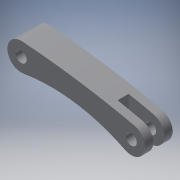
# Autodesk Inventor part: legA_mini
Saved by Autodesk Inventor 2017 (Build 210142000, 142)
## iProperties
Created: 2016-08-26
Part Number: legA_mini
Material: Generic
Document SubType Name: Modeling
Designer: Nic
Density: 1 g/cm^3
Appearance: Default
Author: Nic
Autodesk Inventor part; units mm, degrees
ref_plane "Work Plane1" through (0, 0, 0.75) normal (0, 0, 1) x (1, 0, 0)
ref_plane "YZ Plane" through (0, 0, 0) normal (1, 0, 0) x (0, 1, 0)
ref_plane "XZ Plane" through (0, 0, 0) normal (0, 1, 0) x (-1, 0, 0)
sketch "Sketch1" plane through (0, 0, 0) normal (0, 0, 1) x (1, 0, 0)
  circle A0 centre (0, 0) radius 1
  circle A1 centre (-20, 3) radius 1
  circle A2 centre (-26, 0) radius 1
  arc A3 (-0.9923, -2.2946) -> (1.5226, 1.9828) centre (0, 0) ccw
  arc A4 (-28.125, 3.3889) -> (-24.0417, -3.4878) centre (-26, 0) ccw
  arc A5 (1.5226, 1.9828) -> (-28.125, 3.3889) centre (-14.3125, -18.6387) ccw
  arc A6 (-0.9923, -2.2946) -> (-24.0417, -3.4878) centre (-11.3125, -26.1587) ccw
  dimension "d50" = 2
  dimension "d51" = 3
  dimension "d52" = 20
  dimension "d53" = 6
  dimension "d55" = 2.5
  dimension "d56" = 4
  dimension "d57" = 26
  dimension "d58" = 26
  constraints: 8 point on circle, 7 centre point, 4 tangent, 3 coincident, 2 equal radius, 1 horizontal alignment
  measures "d50" diameter of A0
  measures "d51" vertical distance of A0.centre A1.centre
  measures "d52" horizontal distance of A0.centre A1.centre
  measures "d53" horizontal distance of A2.centre A1.centre
  measures "d55" radius of A3
  measures "d56" radius of A4
  measures "d57" radius of A5
  measures "d58" radius of A6
extrude "Extrusion1" add sketch "Sketch1" along normal blind 5
sketch "Sketch3" plane through (0, 0, 0) normal (0, 1, 0) x (-1, 0, 0)
  line L0 (10, 1.5) -> (45.3794, 1.5)
  line L1 (45.3794, 1.5) -> (45.3794, 3.5)
  line L2 (45.3794, 3.5) -> (10, 3.5)
  line L3 (10, 3.5) -> (10, 1.5)
  line L4 (-0.0755, 0) -> (-0.0755, 5) projected
  point P0 (0, 0)
  dimension "d34" = 1.5
  dimension "d35" = 10
  dimension "d36" = 2
  constraints: 8 end point, 2 parallel, 1 horizontal, 1 perpendicular
  measures "d34" distance from line of L0 point (0, 0)
  measures "d35" distance from line of L3 point (0, 0)
  measures "d36" distance between parallel lines of L2 L0
extrude "Extrusion3" cut sketch "Sketch3" along normal through all both and the other way through all
body "Solid1"
